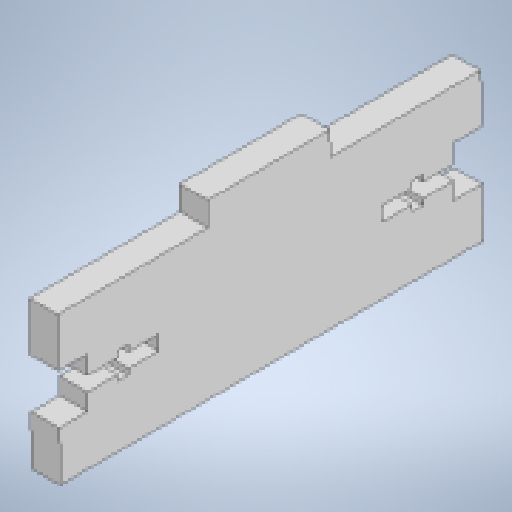
# Autodesk Inventor part: motor1
Saved by Autodesk Inventor 2023.1 (Build 271208000, 208)
## iProperties
Created: 2023-03-16
Part Number: motor1
Material: Типовые
Document SubType Name: Modeling
Designer: User
Density: 1 g/cm^3
Appearance: По умолчанию
Author: User
Autodesk Inventor part; units mm, degrees
ref_plane "РабПлоскость1" through (-327.803629, 8.784154, 215.836479) normal (0, 0, 1) x (1, 0, 0)
sketch "Эскиз1" plane through (-327.803629, 8.784154, 215.836479) normal (0, 0, 1) x (1, 0, 0)
  line L0 (3.114831, 11.166777) -> (2.944416, 21.498705)
  line L1 (2.944416, 21.498705) -> (-3.054768, 21.399754)
  line L2 (-3.054768, 21.399754) -> (-2.884353, 11.067826)
  line L3 (-2.884353, 11.067826) -> (3.114831, 11.166777)
  line L4 (-3.393221, 41.919489) -> (-3.225183, 31.731682)
  line L5 (2.774001, 31.830633) -> (2.605963, 42.01844)
  line L6 (-3.225183, 31.731682) -> (2.774001, 31.830633)
  line L7 (2.605963, 42.01844) -> (-3.393221, 41.919489)
  line L8 (2.774001, 31.830633) -> (2.605963, 42.01844) construction
  line L9 (-3.393221, 41.919489) -> (-3.225183, 31.731682) construction
  line L10 (3.114831, 11.166777) -> (2.944416, 21.498705) construction
  line L11 (-3.054768, 21.399754) -> (-2.884353, 11.067826) construction
  line L12 (6.149374, 48.077701) -> (19.433282, 48.296806) construction
  line L13 (2.605963, 42.01844) -> (6.248325, 42.078517) construction
  point P0 (327.803629, -8.784154)
  dimension "d16" = 6
  constraints: 16 end point
  measures "d16" distance between parallel lines of L13 L12
extrude "Выдавливание1" add sketch "Эскиз1" against normal blind 6
ref_plane "РабПлоскость2" through (-327.498735, 8.403036, 292.836479) normal (0, 0, -1) x (-0.999864, -0.0164918, 0)
sketch "Эскиз2" plane through (-327.498735, 8.403036, 292.836479) normal (0, 0, -1) x (-0.999864, -0.0164918, 0)
  line L0 (-3, 21.833317) -> (3, 21.833317)
  line L1 (3, 21.833317) -> (3, 11.499984)
  line L2 (3, 11.5) -> (-3, 11.5)
  line L3 (-3, 11.499984) -> (-3, 21.833317)
  line L4 (3, 32.16665) -> (-3, 32.16665)
  line L5 (-3, 32.16665) -> (-3, 42.355843)
  line L6 (-3, 42.5) -> (3, 42.5)
  line L7 (3, 42.355843) -> (3, 32.16665)
  line L8 (-3, 11.499984) -> (-3, 21.833317) construction
  line L9 (3, 21.833317) -> (3, 11.499984) construction
  line L10 (-3, 32.16665) -> (-3, 42.355843) construction
  line L11 (3, 42.355843) -> (3, 32.16665) construction
  point P0 (-327.315615, -13.802923)
  constraints: 4 end point
sketch "Эскиз2 outline for Выдавливание2" plane through (-327.498735, 8.403036, 292.836479) normal (0, 0, -1) x (-0.999864, -0.0164918, 0)
  line L0 (3, 32.16665) -> (3, 42.355843)
  line L1 (-3, 32.16665) -> (3, 32.16665)
  line L2 (-3, 42.355843) -> (-3, 32.16665)
  line L3 (3, 42.355843) -> (-3, 42.355843)
  line L4 (-3, 21.833317) -> (-3, 11.499984)
  line L5 (3, 21.833317) -> (-3, 21.833317)
  line L6 (3, 11.499984) -> (3, 21.833317)
  line L7 (-3, 11.499984) -> (3, 11.499984)
extrude "Выдавливание2" add sketch "Эскиз2 outline for Выдавливание2" against normal blind 6
sketch "Эскиз3" plane through (-327.498735, 8.403036, 292.836479) normal (0, 0, -1) x (-0.999864, -0.0164918, 0)
  line L0 (6.642857, 42.355843) -> (3, 42.355843)
  line L1 (-3, 32.166667) -> (-3, 21.833333)
  line L2 (-3, 21.833333) -> (3, 21.833333)
  line L3 (3, 21.833333) -> (3, 32.166667)
  line L4 (3, 32.166667) -> (-3, 32.166667)
  line L5 (-3, 42.355843) -> (3, 42.355843)
  line L6 (3, 42.355843) -> (3, 11.495073)
  line L7 (3, 11.495073) -> (-3, 11.495073)
  line L8 (-3, 11.495073) -> (-3, 42.355843)
  point P0 (-327.315615, -13.802923)
  point P1 (-3, 21.833333)
  point P2 (3, 21.833333)
  point P3 (3, 42.355843)
  constraints: 8 end point, 3 point on line, 2 parallel, 1 horizontal, 1 perpendicular
extrude "Выдавливание3" add sketch "Эскиз3" along normal up to surface (77 mm away)
sketch "Эскиз4" plane through (-331.19685, 50.703643, 209.836479) normal (-0.999864, -0.0164918, 0) x (0, 0, 1)
  line L0 (0, -14) -> (6, -14) construction
  line L1 (0, -17) -> (6, -17) construction
  line L2 (6, -17) -> (6, -14)
  line L3 (6, -14) -> (12.35, -14)
  line L4 (12.35, -14) -> (12.35, -12.75)
  line L5 (12.35, -12.75) -> (14.65, -12.75)
  line L6 (14.65, -12.75) -> (14.65, -14)
  line L7 (14.65, -14) -> (21, -14)
  line L8 (21, -14) -> (21, -17)
  line L9 (21, -17) -> (14.65, -17)
  line L10 (14.65, -17) -> (14.65, -18.25)
  line L11 (14.65, -18.25) -> (12.35, -18.25)
  line L12 (12.35, -18.25) -> (12.35, -17)
  line L13 (12.35, -17) -> (6, -17)
  line L14 (0, -20.522506) -> (0, -30.855843) construction
  line L15 (89, -10.189193) -> (89, 0) construction
  line L16 (0, -30.855843) -> (89, 0) construction
  line L17 (44.5, 0) -> (44.5, -30.855843) construction
  line L18 (89, -14) -> (83, -14) construction
  line L19 (89, -17) -> (83, -17) construction
  line L20 (83, -17) -> (83, -14)
  line L21 (83, -14) -> (76.65, -14)
  line L22 (76.65, -14) -> (76.65, -12.75)
  line L23 (76.65, -12.75) -> (74.35, -12.75)
  line L24 (74.35, -12.75) -> (74.35, -14)
  line L25 (74.35, -14) -> (68, -14)
  line L26 (68, -14) -> (68, -17)
  line L27 (68, -17) -> (74.35, -17)
  line L28 (74.35, -17) -> (74.35, -18.25)
  line L29 (74.35, -18.25) -> (76.65, -18.25)
  line L30 (76.65, -18.25) -> (76.65, -17)
  line L31 (76.65, -17) -> (83, -17)
  point P0 (-209.836479, -56.158766)
  point P1 (44.5, -15.427922)
  dimension "d9" = 2.3
  dimension "d10" = 5.5
  dimension "d11" = 15
  constraints: 62 end point, 14 point on line, 14 symmetric about line, 7 perpendicular, 3 horizontal, 2 collinear, 2 midpoint, 1 horizontal alignment, 1 vertical, 4 other
  measures "d9" distance of L10.end L11.end
  measures "d10" distance between parallel lines of L11 L5
  measures "d11" distance between parallel lines of L8 L2
extrude "Выдавливание4" cut sketch "Эскиз4" against normal blind 6
ref_plane "РабПлоскость3" through (-672.954973, 50.067364, -86.377936) normal (-0.0164918, 0.999864, 0) x (0, 0, 1)
sketch "Эскиз6" plane through (-325.197666, 50.802594, 298.836479) normal (-0.0164918, 0.999864, 0) x (0.999864, 0.0164918, 0)
  line L0 (-6, 89) -> (-6, 0) construction
  line L1 (0, 0) -> (0, 89) construction
  line L2 (-6, 32) -> (0, 32)
  line L3 (0, 32) -> (0, 57)
  line L4 (0, 57) -> (-6, 57)
  line L5 (-6, 57) -> (-6, 32)
  line L6 (0, 89) -> (-6, 89) projected
  line L7 (-3, 89) -> (-3, 57) construction
  line L8 (-3, 32) -> (-3, 0) construction
  line L9 (0, 0) -> (-6, 0) projected
  point P0 (324.315615, 298.836479)
  dimension "d17" = 25
  constraints: 12 end point, 4 midpoint, 3 point on line, 2 parallel, 1 collinear, 1 horizontal, 1 perpendicular
  measures "d17" distance between parallel lines of L2 L4
extrude "Выдавливание6" add sketch "Эскиз6" along normal blind 6
equation "\"d1\" = d0"
equation "\"d3\" = d0"
equation "\"d7\" = d0"
equation "\"d12\" = d3"
equation "\"d0\" = d16"
